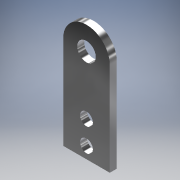
# Autodesk Inventor part: Pulley plate
Saved by Autodesk Inventor 2019.4 (Build 234330000, 330)
## iProperties
Created: 2020-01-24
Part Number: Pulley plate
Material: Aluminum 6061
Document SubType Name: Modeling
Designer: Mark
Mass: 20.0039 g
Surface Area: 34.8531 cm^2
Volume: 7.40884 cm^3
Density: 2.7 g/cm^3
Appearance: Aluminum - Flat
Author: Mark
Autodesk Inventor part; units mm, degrees
ref_plane "YZ Plane" through (0, 0, 0) normal (1, 0, 0) x (0, 1, 0)
ref_plane "XZ Plane" through (0, 0, 0) normal (0, 1, 0) x (-1, 0, 0)
ref_plane "XY Plane" through (0, 0, 0) normal (0, 0, 1) x (1, 0, 0)
sketch "Sketch1" plane through (0, 0, 0) normal (0, 0, 1) x (1, 0, 0)
  line L0 (-10, -11) -> (10, -11)
  line L1 (10, -11) -> (10, 11)
  line L2 (10, 11) -> (0, 11) construction
  line L3 (-10, 11) -> (-10, -11)
  line L4 (-10, -11) -> (10, 11) construction
  line L5 (10, -11) -> (-10, 11) construction
  circle A0 centre (0, -7) radius 2.75
  line L6 (0, 0) -> (0, 20) construction
  line L7 (0, 0) -> (20, 0) construction
  circle A1 centre (0, 20) radius 4
  circle A2 centre (0, 20) radius 8 construction
  arc A3 (10, 20) -> (-10, 20) centre (0, 20) ccw
  line L8 (-10, 11) -> (-10, 20)
  line L9 (10, 20) -> (10, 11)
  line L10 (-10, -11) -> (10, -11)
  circle A4 centre (0, 3.5) radius 2.75
  dimension "d0" = 20
  dimension "d1" = 22
  dimension "d3" = 5.5
  dimension "d4" = 4
  dimension "d8" = 20
  dimension "d9" = 90
  dimension "d10" = 8
  dimension "d11" = 16
  dimension "d12" = 20
  dimension "d23" = 5.5
  dimension "d24" = 10
  dimension "d25" = 5
  constraints: 22 end point, 5 centre point, 3 coincident, 3 horizontal, 3 parallel, 2 midpoint, 2 perpendicular, 2 point on circle, 2 point on line, 1 collinear, 1 tangent, 1 vertical
  measures "d0" distance of L3.start L1.end
  measures "d1" distance of L1.end L0.end
  measures "d3" diameter of A0
  measures "d4" distance from line of L0 A0.centre
  measures "d8" distance of L6.start L6.end
  measures "d9" angle of L7 L6
  measures "d10" diameter of A1
  measures "d11" diameter of A2
  measures "d12" diameter of A3
  measures "d23" diameter of A4
  measures "d24" distance from line of L3 A0.centre
extrude "Extrusion1" add sketch "Sketch1" along normal blind 3
body "Solid1"
